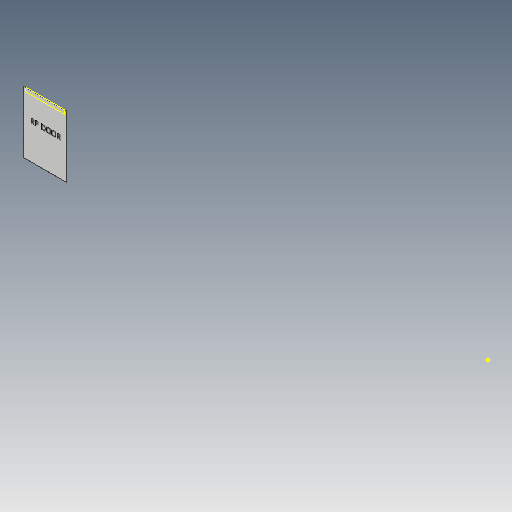
# Autodesk Inventor part: RF_Door
Saved by Autodesk Inventor 2017 (Build 210142000, 142)
## iProperties
Created: 2018-03-27
Part Number: RF_Door
Material: Generic
Document SubType Name: Modeling
Designer: Kathryn Rosie
Density: 1 g/cm^3
Appearance: Default
Author: Kathryn Rosie
Autodesk Inventor part; units mm, degrees
ref_plane "YZ Plane" through (0, 0, 0) normal (1, 0, 0) x (0, 1, 0)
ref_plane "XZ Plane" through (0, 0, 0) normal (0, 1, 0) x (-1, 0, 0)
ref_plane "XY Plane" through (0, 0, 0) normal (0, 0, 1) x (1, 0, 0)
ref_plane "Work Plane1" through (-0.5, 3, -0.5) normal (0, 0, 1) x (1, 0, 0)
sketch "Sketch1" plane through (-0.5, 3, -0.5) normal (0, 0, 1) x (1, 0, 0)
  line L0 (-10391.3804, 103) -> (-10391.3804, -1279) projected
  line L1 (-10304.3804, 106) -> (-9516.7804, 106) projected
  line L2 (-9429.1804, -1279) -> (-9429.1804, 103) projected
  line L3 (-10304.0804, -1275.5) -> (-9516.4804, -1275.5) projected
  line L4 (-10391.3804, 103) -> (-9429.1804, 103)
  line L5 (-9429.1804, 103) -> (-9429.1804, -1279)
  line L6 (-9429.1804, -1279) -> (-10391.3804, -1279)
  line L7 (-10391.3804, -1279) -> (-10391.3804, 103)
  point P0 (0.5, -3)
  constraints: 8 end point, 2 parallel, 1 horizontal, 1 perpendicular
extrude "Extrusion1" add sketch "Sketch1" along normal blind 2
sketch "Sketch2" plane through (-0.5, 3, 1.5) normal (0, 0, 1) x (1, 0, 0)
  line L0 (-10241.6123, -415.187) -> (-9553.7031, -415.187) construction
  line L1 (-9553.7031, -415.187) -> (-9553.7031, -540.2437) construction
  line L2 (-9553.7031, -540.2437) -> (-10241.6123, -540.2437) construction
  line L3 (-10241.6123, -540.2437) -> (-10241.6123, -415.187) construction
  point P0 (0.5, -3)
  constraints: 2 other
body "Solid1"
